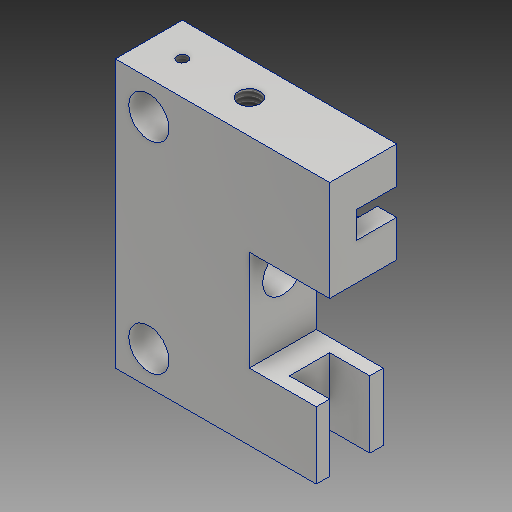
# Autodesk Inventor part: Probenkammer Halter Plus-Seite
Saved by Autodesk Inventor 2017 (Build 210142000, 142)
## iProperties
Part Number: Probenkammer Halter Plus-Seite
Material: Aluminium 6061
Document SubType Name: Modeling
Designer: David Merges
Density: 2.7 g/cm^3
Appearance: Aluminium - flach
Author: David Merges
Autodesk Inventor part; units mm, degrees
ref_plane "YZ Plane" through (0, 0, 0) normal (1, 0, 0) x (0, 1, 0)
ref_plane "XZ Plane" through (0, 0, 0) normal (0, 1, 0) x (-1, 0, 0)
ref_plane "XY Plane" through (0, 0, 0) normal (0, 0, 1) x (1, 0, 0)
sketch "Skizze1" plane through (0, 0, 0) normal (0, 1, 0) x (-1, 0, 0)
  line L0 (5, 20) -> (-15, 20)
  line L1 (-15, 20) -> (-15, -20)
  line L2 (-15, -20) -> (5, -20)
  line L3 (5, -20) -> (5, 20)
  line L4 (0, 15) -> (0, -15) construction
  line L5 (5, 0) -> (0, 0) construction
  circle A0 centre (0, -15) radius 3
  circle A1 centre (0, 15) radius 3
  dimension "d0" = 30
  dimension "d1" = 40
  dimension "d2" = 6
  dimension "d5" = 5
  dimension "d6" = 15
  constraints: 12 end point, 3 coincident, 2 centre point, 2 midpoint, 2 parallel, 2 perpendicular, 1 equal radius, 1 horizontal, 1 vertical
  measures "d0" distance of L4.start L4.end
  measures "d1" distance of L2.end L0.start
  measures "d2" diameter of A0
  measures "d5" distance between parallel lines of L3 L4
  measures "d6" distance between parallel lines of L4 L1
extrude "Extrusion1" add sketch "Skizze1" along normal mid plane 10
sketch "Skizze2" plane through (15, -5, -20) normal (1, 0, 0) x (0, 0, -1)
  circle A0 centre (-20, 5) radius 3
  dimension "d7" = 6
  constraints: 1 centre point, 1 coincident
  measures "d7" diameter of A0
extrude "Extrusion2" cut sketch "Skizze2" against normal through all
sketch "Skizze3" plane through (-5, 5, 20) normal (0, 0, 1) x (1, 0, 0)
  line L0 (20, -10) -> (20, 0) projected
  line L1 (20, -5) -> (15, -5) construction
  point P0 (5, -5)
  dimension "d10" = 5
  constraints: 2 end point, 1 coincident, 1 midpoint, 1 perpendicular
  measures "d10" distance of L1.start L1.end
hole "Bohrung1" at (10, 0, 20) direction (0, 0, -1) diameter 3.242 depth 14 tip angle 118 thread size "M4x0.7" class "6H" standard "ISO Metric profile"
sketch "Skizze4" plane through (-5, 5, 20) normal (0, 0, 1) x (1, 0, 0)
  point P0 (5, -5)
hole "Bohrung2" at (0, 0, 20) direction (0, 0, -1) diameter 1.567 depth 6.3 tip angle 118 thread size "M2x0.4" class "6H" standard "ISO Metric profile"
mirror "Spiegeln2" about plane through (0, 0, 0) normal (0, 0, 1) of "Bohrung2"
sketch "Skizze5" plane through (15, -5, -20) normal (1, 0, 0) x (0, 0, -1)
  circle A0 centre (-20, 5) radius 3 projected
  line L0 (0, 0) -> (0, 10) projected
  line L1 (-40, 10) -> (0, 10) projected
  line L2 (-40, 0) -> (-40, 10) projected
  line L3 (0, 0) -> (-40, 0) projected
  line L4 (-40, 0) -> (-40, 10) projected
  line L5 (-40, 10) -> (0, 10) projected
  line L6 (-40, 0) -> (-25, 0)
  line L7 (-25, 0) -> (-25, 10)
  line L8 (-25, 10) -> (-40, 10)
  line L9 (-40, 10) -> (-40, 0)
  dimension "d25" = 15
  constraints: 8 end point, 2 parallel, 1 horizontal, 1 perpendicular, 1 point on line
  measures "d25" distance between parallel lines of L2 L7
extrude "Extrusion3" add sketch "Skizze5" along normal blind 12 contours L3 L2 L1 L7
sketch "Skizze6" plane through (0, 5, 0) normal (0, 1, 0) x (1, 0, 0)
  circle A0 centre (0, -15) radius 3 projected
  circle A1 centre (0, 15) radius 3 projected
  line L0 (-5, -20) -> (27, -20) projected
  line L1 (27, -5) -> (27, -20) projected
  line L2 (15, -5) -> (27, -5) projected
  line L3 (15, -5) -> (15, 20) projected
  line L4 (15, 20) -> (-5, 20) projected
  line L5 (-5, 20) -> (-5, -20) projected
  line L6 (15, -5) -> (15, 20) construction
  circle A2 centre (19.5, -12.5) radius 5.05
  line L7 (27, -5) -> (27, -20) projected
  line L8 (27, -12.5) -> (19.5, -12.5) construction
  line L9 (25.2991, -5) -> (25.2991, -12.5) construction
  point P0 (0, 0)
  dimension "d28" = 10.1
  constraints: 4 end point, 2 perpendicular, 2 point on line, 1 centre point, 1 horizontal, 1 midpoint
  measures "d28" diameter of A2
extrude "Extrusion4" cut sketch "Skizze6" against normal blind 6 contours A2
sketch "Skizze7" plane through (0, 5, 0) normal (0, 1, 0) x (1, 0, 0)
  circle A0 centre (19.5, -12.5) radius 5.05 projected
  circle A1 centre (0, -15) radius 3 projected
  circle A2 centre (0, 15) radius 3 projected
  line L0 (-5, -20) -> (27, -20) projected
  line L1 (27, -5) -> (27, -20) projected
  line L2 (15, -5) -> (27, -5) projected
  line L3 (15, -5) -> (15, 20) projected
  line L4 (15, 20) -> (-5, 20) projected
  line L5 (-5, 20) -> (-5, -20) projected
  line L6 (27, -5) -> (27, -20) projected
  line L7 (27, -14.5) -> (17.9872, -14.5)
  line L8 (17.9872, -14.5) -> (17.9872, -10.5)
  line L9 (17.9872, -10.5) -> (27, -10.5)
  line L10 (27, -10.5) -> (27, -14.5)
  point P0 (0, 0)
  point P1 (27, -12.5)
  dimension "d37" = 4
  constraints: 8 end point, 2 midpoint, 2 parallel, 1 horizontal, 1 perpendicular, 1 point on line
  measures "d37" distance between parallel lines of L7 L9
sketch "Skizze8" plane through (15, -5, -20) normal (1, 0, 0) x (0, 0, -1)
  line L0 (-25, 10) -> (-25, 0) projected
  line L1 (0, 0) -> (-25, 0) projected
  line L2 (0, 0) -> (0, 10) projected
  line L3 (-25, 10) -> (0, 10) projected
  circle A0 centre (-20, 5) radius 3 projected
  line L4 (0, 0) -> (-10, 0)
  line L5 (-10, 0) -> (-10, 10)
  line L6 (-10, 10) -> (0, 10)
  line L7 (0, 10) -> (0, 0)
  dimension "d31" = 10
  constraints: 8 end point, 2 parallel, 1 horizontal, 1 perpendicular, 1 point on line
  measures "d31" distance of L5.end L6.end
extrude "Extrusion5" add sketch "Skizze8" along normal blind 10 contours L3 L2 L1 L5
sketch "Skizze9" plane through (25, -5, -20) normal (1, 0, 0) x (0, 0, -1)
  line L0 (0, 0) -> (0, 10) projected
  line L1 (0, 10) -> (-10, 10) projected
  line L2 (-10, 10) -> (-10, 0) projected
  line L3 (-10, 0) -> (0, 0) projected
  line L4 (-10, 2) -> (0, 2)
  line L5 (0, 2) -> (0, 8)
  line L6 (0, 8) -> (-10, 8)
  line L7 (-10, 8) -> (-10, 2)
  point P0 (-20, 5)
  point P1 (0, 5)
  dimension "d34" = 6
  constraints: 8 end point, 2 midpoint, 2 parallel, 2 point on line, 1 horizontal, 1 perpendicular
  measures "d34" distance between parallel lines of L6 L4
extrude "Extrusion6" cut sketch "Skizze9" against normal blind 6 contours L4 L2 L6 L0
extrude "Extrusion7" cut sketch "Skizze7" against normal up to surface (6 mm away) contours A0 L7 L8 L9 | A0 L9 L1 L7 picked at (20.1748, -12.5)
